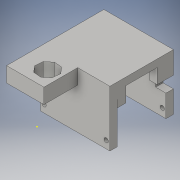
# Autodesk Inventor part: right side
Saved by Autodesk Inventor 2016 (Build 200138000, 138)
## iProperties
Created: 2015-04-28
Part Number: right side
Material: Generic
Document SubType Name: Modeling
Designer: Jacob Kennedy
Density: 1 g/cm^3
Appearance: Default
Author: Jacob Kennedy
Autodesk Inventor part; units mm, degrees
ref_plane "YZ Plane" through (0, 0, 0) normal (1, 0, 0) x (0, 1, 0)
ref_plane "XZ Plane" through (0, 0, 0) normal (0, 1, 0) x (-1, 0, 0)
ref_plane "XY Plane" through (0, 0, 0) normal (0, 0, 1) x (1, 0, 0)
sketch "Sketch1" plane through (0, 0, 0) normal (0, 1, 0) x (-1, 0, 0)
  line L0 (-21.8816, 15.8348) -> (-21.8816, -13.2164)
  line L1 (-21.8816, -13.2164) -> (10.224, -13.2164)
  line L2 (10.224, 15.8348) -> (0.9022, 15.8348)
  line L3 (10.224, -13.2164) -> (10.224, 15.8348)
  line L4 (0.9022, 15.8348) -> (-21.8816, 15.8348)
  line L5 (-21.8816, 15.8348) -> (-21.8816, 9.4848)
  line L6 (-21.8816, -13.2164) -> (0.9022, -13.2164)
  line L7 (-2.558, -2.8836) -> (-7.7902, -7.2872)
  line L8 (-7.7902, -7.2872) -> (-14.6037, -6.7012)
  line L9 (-14.6037, -6.7012) -> (-19.0073, -1.469)
  line L10 (-19.0073, -1.469) -> (-18.4213, 5.3445)
  line L11 (-18.4213, 5.3445) -> (-13.1891, 9.7481)
  line L12 (-13.1891, 9.7481) -> (-6.3756, 9.1621)
  line L13 (-6.3756, 9.1621) -> (-1.972, 3.9299)
  line L14 (-1.972, 3.9299) -> (-2.558, -2.8836)
  line L15 (10.224, -13.2164) -> (-49.5803, -13.2164)
  line L16 (-49.5803, -13.2164) -> (-49.5803, -19.5664)
  line L17 (-49.5803, -19.5664) -> (10.224, -19.5664)
  line L18 (10.224, -19.5664) -> (10.224, -13.2164)
  line L19 (10.224, -19.5664) -> (-49.5803, -19.5664)
  line L20 (-49.5803, -19.5664) -> (-49.5803, -74.1256)
  line L21 (-49.5803, -74.1256) -> (10.224, -74.1256)
  line L22 (10.224, -74.1256) -> (10.224, -19.5664)
  line L23 (10.224, -22.2907) -> (3.874, -22.2907)
  line L24 (3.874, -22.2907) -> (3.874, -35.7778)
  line L25 (3.874, -35.7778) -> (10.224, -35.7778)
  line L26 (10.224, -35.7778) -> (10.224, -22.2907)
  line L27 (-49.5803, -22.2907) -> (-43.2303, -22.2907)
  line L28 (-43.2303, -22.2907) -> (-43.2303, -35.7778)
  line L29 (-43.2303, -35.7778) -> (-49.5803, -35.7778)
  line L30 (-49.5803, -35.7778) -> (-49.5803, -22.2907)
  line L31 (-49.5803, -74.1256) -> (10.224, -74.1256)
  line L32 (10.224, -74.1256) -> (10.224, -61.4256)
  line L33 (10.224, -61.4256) -> (-49.5803, -61.4256)
  line L34 (-49.5803, -61.4256) -> (-49.5803, -74.1256)
  line L35 (10.224, -19.5664) -> (3.874, -19.5664)
  line L36 (3.874, -19.5664) -> (3.874, -74.1256)
  line L37 (3.874, -74.1256) -> (10.224, -74.1256)
  line L38 (10.224, -74.1256) -> (10.224, -19.5664)
  line L39 (-49.5803, -74.1256) -> (-43.2303, -74.1256)
  line L40 (-43.2303, -74.1256) -> (-43.2303, -19.5664)
  line L41 (-43.2303, -19.5664) -> (-49.5803, -19.5664)
  line L42 (-49.5803, -19.5664) -> (-49.5803, -74.1256)
  line L43 (10.224, -46.846) -> (3.874, -46.846)
  line L44 (3.874, -46.846) -> (3.874, -58.2621)
  line L45 (3.874, -58.2621) -> (10.224, -58.2621)
  line L46 (10.224, -58.2621) -> (10.224, -46.846)
  line L47 (-43.2303, -46.846) -> (-49.5803, -46.846)
  line L48 (-49.5803, -46.846) -> (-49.5803, -58.2621)
  line L49 (-49.5803, -58.2621) -> (-43.2303, -58.2621)
  line L50 (-43.2303, -58.2621) -> (-43.2303, -46.846)
  point P0 (0, 0)
  point P1 (-10.4897, 1.2304)
  dimension "d0" = 29.0512
  dimension "d1" = 32.1056
  dimension "d5" = 16.51
  dimension "d6" = 6.35
  dimension "d8" = 59.8043
  dimension "d9" = 54.5592
  dimension "d10" = 59.8043
  dimension "d11" = 6.35
  dimension "d12" = 12.7
  dimension "d13" = 6.35
  dimension "d14" = 47.1043
  dimension "d15" = 41.8592
  dimension "d16" = 6.35
  dimension "d17" = 6.35
  constraints: 102 end point, 18 parallel, 12 horizontal, 12 point on line, 11 perpendicular, 2 midpoint, 17 other
  measures "d0" distance of L1.end L2.start
  measures "d1" distance of L0.end L1.end
  measures "d5" distance between parallel lines of L8 L12
  measures "d6" distance of L15.end L16.end
  measures "d8" distance of L1.end L15.end
  measures "d9" distance of L21.end L17.end
  measures "d10" distance of L20.end L21.end
  measures "d11" distance between parallel lines of L22 L36
  measures "d12" distance between parallel lines of L21 L33
  measures "d13" distance between parallel lines of L40 L42
  measures "d14" distance between parallel lines of L40 L36
  measures "d15" distance between parallel lines of L33 L19
  measures "d16" distance of L24.end L25.end
  measures "d17" distance of L28.end L29.end
extrude "Extrusion1" add sketch "Sketch1" along normal blind 12.9921 contours L4 L2 L3 L1 L0
sketch "Sketch2" plane through (0, 0, 0) normal (0, -1, 0) x (1, 0, 0)
  line L0 (-10.224, -13.2164) -> (49.593, -13.2164)
  line L1 (49.593, -13.2164) -> (49.593, -19.5664)
  line L2 (49.593, -19.5664) -> (-10.224, -19.5664)
  line L3 (-10.224, -19.5664) -> (-10.224, -13.2164)
  point P0 (0, 0)
  dimension "d20" = 6.35
  dimension "d21" = 59.817
  constraints: 8 end point, 2 parallel, 1 horizontal, 1 perpendicular
  measures "d20" distance of L2.end L0.start
  measures "d21" distance of L1.end L2.end
extrude "Extrusion2" add sketch "Sketch2" along normal blind 35.2679
sketch "Sketch3" plane through (0, 0, 0) normal (0, 1, 0) x (1, 0, 0)
  line L0 (21.8816, 13.2164) -> (-10.224, 13.2164) projected
  line L1 (-10.224, 19.5664) -> (49.593, 19.5664) projected
  line L2 (-10.224, 13.2164) -> (49.593, 13.2164)
  line L3 (49.593, 13.2164) -> (49.593, 19.5664)
  line L4 (49.593, 19.5664) -> (-10.224, 19.5664)
  line L5 (-10.224, 19.5664) -> (-10.224, 13.2164)
  point P0 (0, 0)
  constraints: 8 end point, 2 parallel, 1 horizontal, 1 perpendicular
extrude "Extrusion3" add sketch "Sketch3" along normal blind 12.9921
sketch "Sketch4" plane through (49.593, -35.2679, -19.5664) normal (0, 0, -1) x (-1, 0, 0)
  line L0 (59.817, 48.26) -> (27.7114, 48.26) projected
  line L1 (0, 0) -> (0, 48.26) projected
  line L2 (59.817, 48.26) -> (0, 48.26)
  line L3 (0, 48.26) -> (0, 35.2679)
  line L4 (0, 35.2679) -> (59.817, 35.2679)
  line L5 (59.817, 35.2679) -> (59.817, 48.26)
  point P0 (49.593, 35.2679)
  dimension "d26" = 59.817
  dimension "d27" = 12.9921
  constraints: 8 end point, 2 parallel, 1 horizontal, 1 perpendicular, 1 point on line
  measures "d26" distance of L3.end L4.end
  measures "d27" distance of L4.end L0.start
extrude "Extrusion4" add sketch "Sketch4" along normal blind 48.26
sketch "Sketch5" plane through (-10.224, 0, -19.5664) normal (0, -1, 0) x (1, 0, 0)
  line L0 (0, 35.4013) -> (0, -48.26) projected
  line L1 (59.817, 6.35) -> (59.817, -48.26) projected
  line L2 (0, -48.26) -> (59.817, -48.26)
  line L3 (59.817, -48.26) -> (59.817, -41.8786)
  line L4 (59.817, -41.8786) -> (0, -41.8786)
  line L5 (0, -41.8786) -> (0, -48.26)
  point P0 (10.224, 19.5664)
  constraints: 8 end point, 2 parallel, 1 horizontal, 1 perpendicular, 1 point on line
extrude "Extrusion5" add sketch "Sketch5" along normal blind 35.2679
sketch "Sketch6" plane through (-10.224, 0, -19.5664) normal (0, -1, 0) x (1, 0, 0)
  line L0 (0, 0) -> (0, -41.8786) projected
  line L1 (0, -41.8786) -> (6.35, -41.8786)
  line L2 (6.35, -41.8786) -> (6.35, -34.2586)
  line L3 (6.35, -34.2586) -> (0, -34.2586)
  line L4 (0, -34.2586) -> (0, -41.8786)
  line L5 (0, -7.2782) -> (6.35, -7.2782)
  line L6 (6.35, -7.2782) -> (6.35, -0.0002)
  line L7 (6.35, -0.0002) -> (0, -0.0002)
  line L8 (0, -0.0002) -> (0, -7.2782)
  line L9 (59.817, 6.35) -> (59.817, -48.26) projected
  line L10 (59.817, -41.8786) -> (53.467, -41.8786)
  line L11 (53.467, -41.8786) -> (53.467, -34.2586)
  line L12 (53.467, -34.2586) -> (59.817, -34.2586)
  line L13 (59.817, -34.2586) -> (59.817, -41.8786)
  line L14 (59.817, -0.0002) -> (53.467, -0.0002)
  line L15 (53.467, -0.0002) -> (53.467, -7.2782)
  line L16 (53.467, -7.2782) -> (59.817, -7.2782)
  line L17 (59.817, -7.2782) -> (59.817, -0.0002)
  point P0 (10.224, 19.5664)
  constraints: 32 end point, 9 point on line, 8 parallel, 4 horizontal, 4 perpendicular
extrude "Extrusion6" add sketch "Sketch6" along normal blind 6.35
sketch "Sketch7" plane through (49.593, -35.2679, -67.8264) normal (0, 0, -1) x (-1, 0, 0)
  line L0 (27.7114, 48.26) -> (0, 48.26) projected
  line L1 (0, 0) -> (59.817, 0) projected
  line L2 (0, 48.26) -> (8.89, 48.26)
  line L3 (8.89, 48.26) -> (8.89, 0)
  line L4 (8.89, 0) -> (0, 0)
  line L5 (0, 0) -> (0, 48.26)
  line L6 (0, 48.26) -> (8.89, 48.26)
  line L7 (8.89, 48.26) -> (8.89, 29.21)
  line L8 (8.89, 29.21) -> (0, 29.21)
  line L9 (0, 29.21) -> (0, 48.26)
  line L10 (0, 28.9179) -> (0, 0) projected
  line L11 (0, 0) -> (8.89, 0)
  line L12 (8.89, 0) -> (8.89, 19.05)
  line L13 (8.89, 19.05) -> (0, 19.05)
  line L14 (0, 19.05) -> (0, 0)
  line L15 (8.89, 29.21) -> (0, 29.21)
  line L16 (0, 29.21) -> (0, 19.05)
  line L17 (0, 19.05) -> (8.89, 19.05)
  line L18 (8.89, 19.05) -> (8.89, 29.21)
  point P0 (49.593, 35.2679)
  dimension "d39" = 8.89
  dimension "d40" = 19.05
  dimension "d41" = 19.05
  constraints: 32 end point, 8 parallel, 4 horizontal, 4 perpendicular, 3 point on line
  measures "d39" distance of L0.end L2.end
  measures "d40" distance of L6.end L7.end
  measures "d41" distance of L11.end L12.end
extrude "Extrusion7" cut sketch "Sketch7" along normal mid plane 42.8625 contours L3 L13 L5 L8
sketch "Sketch8" plane through (-10.224, 0, -19.5664) normal (0, -1, 0) x (1, 0, 0)
  line L0 (6.35, -41.8786) -> (6.35, -34.2586) projected
  line L1 (6.35, -41.8786) -> (53.467, -41.8786)
  line L2 (53.467, -41.8786) -> (53.467, -34.2586)
  line L3 (53.467, -34.2586) -> (6.35, -34.2586)
  line L4 (6.35, -34.2586) -> (6.35, -41.8786)
  line L5 (0, -34.2586) -> (6.35, -34.2586) projected
  line L6 (59.817, -7.2782) -> (59.817, -0.0002) projected
  line L7 (0, -34.2586) -> (59.817, -34.2586)
  line L8 (59.817, -34.2586) -> (59.817, -7.2782)
  line L9 (59.817, -7.2782) -> (0, -7.2782)
  line L10 (0, -7.2782) -> (0, -34.2586)
  line L11 (53.467, -0.0002) -> (53.467, -7.2782) projected
  line L12 (6.35, -7.2782) -> (53.467, -7.2782)
  line L13 (53.467, -7.2782) -> (53.467, -0.0002)
  line L14 (53.467, -0.0002) -> (6.35, -0.0002)
  line L15 (6.35, -0.0002) -> (6.35, -7.2782)
  point P0 (10.224, 19.5664)
  constraints: 24 end point, 6 parallel, 3 horizontal, 3 perpendicular, 2 point on line
extrude "Extrusion8" cut sketch "Sketch8" against normal blind 6.6421
sketch "Sketch9" plane through (-10.224, -35.2679, -19.5664) normal (0, -1, 0) x (1, 0, 0)
  point P0 (10.224, 19.5664)
sketch "Sketch10" plane through (49.593, -35.2679, -67.8264) normal (0, 0, -1) x (-1, 0, 0)
  line L0 (59.817, 0) -> (0, 0) projected
  line L1 (0, 0) -> (0, 48.26) projected
  circle A0 centre (3.175, 6.5024) radius 1.8796
  circle A1 centre (56.642, 6.5024) radius 1.8796
  point P0 (49.593, 35.2679)
  constraints: 2 centre point
extrude "Extrusion9" cut sketch "Sketch10" along normal mid plane 147.9296
body "Solid1"
